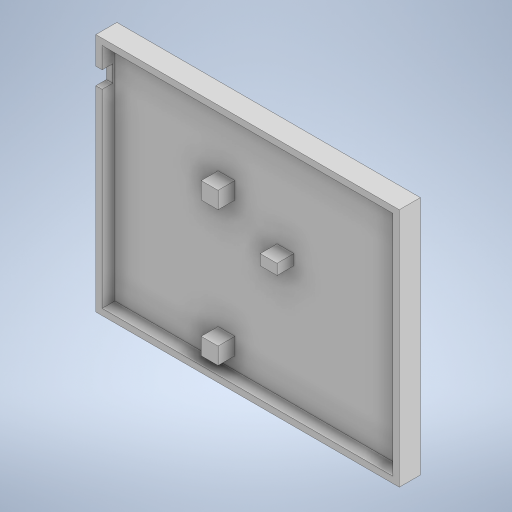
# Autodesk Inventor part: support
Saved by Autodesk Inventor 2024 (Build 280153000, 153)
## iProperties
Created: 2024-03-12
Part Number: support
Material: Générique
Document SubType Name: Modeling
Designer: phaly
Density: 1 g/cm^3
Appearance: Par défaut
Author: phaly
Autodesk Inventor part; units mm, degrees
ref_plane "YZ Plane" through (0, 0, 0) normal (1, 0, 0) x (0, 1, 0)
ref_plane "XZ Plane" through (0, 0, 0) normal (0, 1, 0) x (-1, 0, 0)
ref_plane "XY Plane" through (0, 0, 0) normal (0, 0, 1) x (1, 0, 0)
sketch "Esquisse1" plane through (0, 0, 0) normal (0, 0, 1) x (1, 0, 0)
  line L0 (0, 114) -> (144, 114)
  line L1 (144, 114) -> (144, 0)
  line L2 (144, 0) -> (0, 0)
  line L3 (0, 0) -> (0, 114)
  line L4 (3, 111) -> (141, 111)
  line L5 (141, 111) -> (141, 3)
  line L6 (141, 3) -> (3, 3)
  line L7 (3, 3) -> (3, 111)
  line L8 (0, -22.8) -> (0, 136.8) projected
  line L9 (-28.8, 0) -> (172.8, 0) projected
  point P0 (0, 0)
  dimension "d0" = 114
  dimension "d1" = 144
  dimension "d2" = 3
  dimension "d3" = 3
  dimension "d4" = 3
  dimension "d5" = 3
  constraints: 16 end point, 4 parallel, 2 collinear, 2 horizontal, 2 perpendicular
  measures "d0" distance of L2.end L0.start
  measures "d1" distance of L0.start L0.end
  measures "d2" distance between parallel lines of L0 L4
  measures "d3" distance between parallel lines of L2 L6
  measures "d4" distance between parallel lines of L3 L7
  measures "d5" distance between parallel lines of L1 L5
extrude "Extrusion1" add sketch "Esquisse1" along normal blind 10
sketch "Esquisse2" plane through (0, 0, 0) normal (0, 0, -1) x (-1, 0, 0)
  line L0 (0, 114) -> (-144, 114)
  line L1 (-144, 114) -> (-144, 0)
  line L2 (-144, 0) -> (0, 0)
  line L3 (0, 0) -> (0, 114)
  line L4 (0, 114) -> (0, 0) projected
  line L5 (-144, 114) -> (0, 114) projected
  line L6 (0, 0) -> (-144, 0) projected
  line L7 (-144, 0) -> (-144, 114) projected
  constraints: 8 end point, 4 collinear, 2 parallel, 1 horizontal, 1 perpendicular
extrude "Extrusion2" add sketch "Esquisse2" against normal blind 4
sketch "Esquisse3" plane through (0, 0, 4) normal (0, 0, 1) x (1, 0, 0)
  line L0 (52, 81) -> (60, 81)
  line L1 (60, 81) -> (60, 73)
  line L2 (60, 73) -> (52, 73)
  line L3 (52, 73) -> (52, 81)
  line L4 (52, 17) -> (60, 17)
  line L5 (60, 17) -> (60, 9)
  line L6 (60, 9) -> (52, 9)
  line L7 (52, 9) -> (52, 17)
  line L8 (80, 65) -> (88, 65)
  line L9 (88, 65) -> (88, 60)
  line L10 (88, 60) -> (80, 60)
  line L11 (80, 60) -> (80, 65)
  line L12 (141, 111) -> (141, 3) projected
  line L13 (141, 3) -> (3, 3) projected
  point P0 (0, 0)
  dimension "d10" = 8
  dimension "d11" = 8
  dimension "d12" = 8
  dimension "d13" = 8
  dimension "d14" = 8
  dimension "d15" = 5
  dimension "d16" = 89
  dimension "d17" = 61
  dimension "d18" = 6
  dimension "d19" = 56
  dimension "d20" = 8
  constraints: 24 end point, 6 parallel, 3 horizontal, 3 perpendicular, 1 collinear
  measures "d10" distance of L0.start L0.end
  measures "d11" distance of L2.end L0.start
  measures "d12" distance of L5.end L6.end
  measures "d13" distance of L6.end L4.start
  measures "d14" distance of L8.start L8.end
  measures "d15" distance of L10.end L8.start
  measures "d16" distance between parallel lines of L12 L7
  measures "d17" distance between parallel lines of L12 L11
  measures "d18" distance between parallel lines of L13 L6
  measures "d19" distance between parallel lines of L2 L4
  measures "d20" distance between parallel lines of L8 L2
extrude "Extrusion3" add sketch "Esquisse3" along normal blind 8
sketch "Esquisse5" plane through (0, 0, 0) normal (-1, 0, 0) x (0, 0, 1)
  line L0 (10, 101) -> (5, 101)
  line L1 (5, 101) -> (5, 93)
  line L2 (5, 93) -> (10, 93)
  line L3 (10, 93) -> (10, 101)
  line L4 (0, 114) -> (10, 114) projected
  line L5 (10, 114) -> (10, 0) projected
  point P0 (0, 0)
  dimension "d23" = 13
  dimension "d24" = 8
  dimension "d25" = 5
  constraints: 8 end point, 2 parallel, 1 collinear, 1 horizontal, 1 perpendicular
  measures "d23" distance between parallel lines of L4 L0
  measures "d24" distance of L2.end L0.start
  measures "d25" distance between parallel lines of L5 L1
extrude "Extrusion4" cut sketch "Esquisse5" against normal blind 8
equation "\"d3\" = d2"
equation "\"d4\" = d3"
equation "\"d5\" = d4"
equation "\"d11\" = d10"
equation "\"d12\" = d10"
equation "\"d13\" = d12"
equation "\"d14\" = d10"
